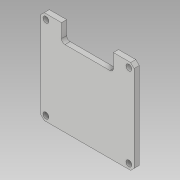
# Autodesk Inventor part: bearing_mount_part_1
Saved by Autodesk Inventor 2017 (Build 210142000, 142)
## iProperties
Part Number: bearing_mount_part_1
Material: Aluminium 6061
Document SubType Name: Modeling
Designer: Max
Density: 2.7 g/cm^3
Appearance: Vorgabe
Mass: 14.2204 g
Surface Area: 58.1145 cm^2
Volume: 5.2668 cm^3
Author: Max
Autodesk Inventor part; units mm, degrees
ref_plane "YZ Plane" through (0, 0, 0) normal (1, 0, 0) x (0, 1, 0)
ref_plane "XZ Plane" through (0, 0, 0) normal (0, 1, 0) x (-1, 0, 0)
ref_plane "XY Plane" through (0, 0, 0) normal (0, 0, 1) x (1, 0, 0)
sketch "Skizze1" plane through (0, 0, 0) normal (0, 1, 0) x (-1, 0, 0)
  line L0 (-27, 27) -> (27, 27)
  line L1 (27, 27) -> (27, -27)
  line L2 (27, -27) -> (-27, -27)
  line L3 (-27, -27) -> (-27, 27)
  line L4 (-27, 27) -> (27, -27) construction
  line L5 (27, 27) -> (-27, -27) construction
  point P0 (0, 0)
  dimension "d0" = 54
  dimension "d1" = 54
  constraints: 12 end point, 2 midpoint, 2 parallel, 1 horizontal, 1 perpendicular
  measures "d0" distance of L1.end L2.end
  measures "d1" distance of L0.end L1.end
extrude "Extrusion1" add sketch "Skizze1" along normal blind 3
chamfer "Fase1" distance 2 angle 45 4 edges at (27, 1.5, 27) (27, 1.5, -27) (-27, 1.5, 27) (-27, 1.5, -27)
sketch "Skizze2" plane through (0, 3, 0) normal (0, 1, 0) x (1, 0, 0)
  circle A0 centre (0, 0) radius 11
  dimension "d7" = 22
  constraints: 1 centre point, 1 coincident
  measures "d7" diameter of A0
extrude "Extrusion2" [suppressed]
sketch "Skizze4" plane through (0, 3, 0) normal (0, 1, 0) x (1, 0, 0)
  line L0 (-24, -24) -> (24, -24)
  line L1 (24, -24) -> (24, 24)
  line L2 (24, 24) -> (-24, 24)
  line L3 (-24, 24) -> (-24, -24)
  line L4 (-24, -24) -> (24, 24) construction
  line L5 (24, -24) -> (-24, 24) construction
  point P0 (0, 0)
  dimension "d13" = 48
  dimension "d14" = 48
  constraints: 12 end point, 2 midpoint, 2 parallel, 1 horizontal, 1 perpendicular
  measures "d13" distance of L1.end L2.end
  measures "d14" distance of L0.end L1.end
hole "Bohrung1" at (24, 3, -24) at (24, 3, 24) at (-24, 3, 24) at (-24, 3, -24) direction (0, -1, 0) diameter 3.4 end through all clearance for "Inbusschraube ISO 4762" size "M3" standard "ISO"
sketch "Skizze5" plane through (0, 0, 0) normal (0, -1, 0) x (1, 0, 0)
  line L0 (15, 37) -> (-15, 37)
  line L1 (-15, 37) -> (-15, 17)
  line L2 (-15, 17) -> (15, 17)
  line L3 (15, 17) -> (15, 37)
  line L4 (-25, 27) -> (25, 27) projected
  line L5 (15, 37) -> (-15, 17) construction
  line L6 (-15, 37) -> (15, 17) construction
  point P0 (0, 0)
  point P1 (0, 27)
  dimension "d22" = 30
  dimension "d23" = 10
  constraints: 12 end point, 3 midpoint, 2 parallel, 1 horizontal, 1 perpendicular
  measures "d22" distance of L0.start L0.end
  measures "d23" distance between parallel lines of L4 L2
extrude "Extrusion4" cut sketch "Skizze5" against normal blind 3
fillet "Rundung1" radius 2 2 edges at (-15, 1.5, 17) (15, 1.5, 17)
